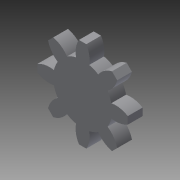
# Autodesk Inventor part: Planet
Saved by Autodesk Inventor 2013 (Build 170138000, 138)
## iProperties
Created: 2014-02-12
Part Number: Planet
Material: Generic
Document SubType Name: Modeling
Designer: robotics
Density: 1 g/cm^3
Author: robotics
Autodesk Inventor part; units mm, degrees
ref_plane "YZ Plane" through (0, 0, 0) normal (1, 0, 0) x (0, 1, 0)
ref_plane "XZ Plane" through (0, 0, 0) normal (0, 1, 0) x (-1, 0, 0)
ref_plane "XY Plane" through (0, 0, 0) normal (0, 0, 1) x (1, 0, 0)
sketch "Sketch2" plane through (0, 0, 0) normal (0, 0, 1) x (1, 0, 0)
  line L0 (0, 0) -> (0, 8.357) construction
  line L1 (0, 0) -> (2.8603, 0) construction
  arc A0 (-0.3969, 4.8591) -> (-0.71, 3.0831) centre (1.785, 3.5588) ccw
  arc A1 (0.71, 3.0831) -> (0.3969, 4.8591) centre (-1.785, 3.5588) ccw
  line L2 (0.3969, 4.8591) -> (-0.3969, 4.8591)
  line L3 (-0.71, 3.0831) -> (0.71, 3.0831) construction
  arc A2 (0.71, 3.0831) -> (0.3969, 4.8591) centre (-1.785, 3.5588) ccw
  line L4 (0.3969, 4.8591) -> (-0.3969, 4.8591)
  arc A3 (-0.3969, 4.8591) -> (-0.71, 3.0831) centre (1.785, 3.5588) ccw
  line L5 (0.3969, 4.8591) -> (0.71, 3.0831) construction
  arc A4 (-1.678, 2.6822) -> (-3.1553, 3.7166) centre (-3.7786, 1.2542) ccw
  line L6 (-3.1553, 3.7166) -> (-3.7166, 3.1553)
  arc A5 (-3.7166, 3.1553) -> (-2.6822, 1.678) centre (-1.2542, 3.7786) ccw
  arc A6 (-3.0831, 0.71) -> (-4.8591, 0.3969) centre (-3.5588, -1.785) ccw
  line L7 (-4.8591, 0.3969) -> (-4.8591, -0.3969)
  arc A7 (-4.8591, -0.3969) -> (-3.0831, -0.71) centre (-3.5588, 1.785) ccw
  arc A8 (-2.6822, -1.678) -> (-3.7166, -3.1553) centre (-1.2542, -3.7786) ccw
  line L8 (-3.7166, -3.1553) -> (-3.1553, -3.7166)
  arc A9 (-3.1553, -3.7166) -> (-1.678, -2.6822) centre (-3.7786, -1.2542) ccw
  arc A10 (-0.71, -3.0831) -> (-0.3969, -4.8591) centre (1.785, -3.5588) ccw
  line L9 (-0.3969, -4.8591) -> (0.3969, -4.8591)
  arc A11 (0.3969, -4.8591) -> (0.71, -3.0831) centre (-1.785, -3.5588) ccw
  arc A12 (1.678, -2.6822) -> (3.1553, -3.7166) centre (3.7786, -1.2542) ccw
  line L10 (3.1553, -3.7166) -> (3.7166, -3.1553)
  arc A13 (3.7166, -3.1553) -> (2.6822, -1.678) centre (1.2542, -3.7786) ccw
  arc A14 (3.0831, -0.71) -> (4.8591, -0.3969) centre (3.5588, 1.785) ccw
  line L11 (4.8591, -0.3969) -> (4.8591, 0.3969)
  arc A15 (4.8591, 0.3969) -> (3.0831, 0.71) centre (3.5588, -1.785) ccw
  arc A16 (2.6822, 1.678) -> (3.7166, 3.1553) centre (1.2542, 3.7786) ccw
  line L12 (3.7166, 3.1553) -> (3.1553, 3.7166)
  arc A17 (3.1553, 3.7166) -> (1.678, 2.6822) centre (3.7786, 1.2542) ccw
  line L13 (-1.678, 2.6822) -> (-0.71, 3.0831) construction
  arc A18 (-0.71, 3.0831) -> (-1.678, 2.6822) centre (0, 0) ccw
  arc A19 (1.678, 2.6822) -> (0.71, 3.0831) centre (0, 0) ccw
  arc A20 (3.0831, 0.71) -> (2.6822, 1.678) centre (0, 0) ccw
  arc A21 (2.6822, -1.678) -> (3.0831, -0.71) centre (0, 0) ccw
  arc A22 (0.71, -3.0831) -> (1.678, -2.6822) centre (0, 0) ccw
  arc A23 (-1.678, -2.6822) -> (-0.71, -3.0831) centre (0, 0) ccw
  arc A24 (-2.6822, 1.678) -> (-3.0831, 0.71) centre (0, 0) ccw
  arc A25 (-3.0831, -0.71) -> (-2.6822, -1.678) centre (0, 0) ccw
  point P0 (0, 4.8591)
  point P1 (-3.4359, 3.4359)
  point P2 (-4.8591, 0)
  point P3 (-3.4359, -3.4359)
  point P4 (0, -4.8591)
  point P5 (3.4359, -3.4359)
  point P6 (4.8591, 0)
  point P7 (3.4359, 3.4359)
  dimension "d11" = 0.7937
  dimension "d13" = 2.54
  dimension "d14" = 80
  dimension "d15" = 1.8034
  dimension "d18" = 360
  dimension "d20" = 1.0477
  constraints: 52 point on circle, 28 end point, 26 centre point, 2 concentric, 1 coincident, 1 collinear, 1 horizontal, 1 horizontal alignment, 1 midpoint, 1 parallel, 1 perpendicular, 1 vertical, 1 vertical alignment, 81 other
  measures "d11" distance of L2.start L2.end
  measures "d13" radius of A1
  measures "d14" angle of L1 L5
  measures "d15" distance of L2.start L3.end
  measures "d20" distance of L3.start L13.start
extrude "Extrusion2" add sketch "Sketch2" along normal blind 1.5875
body "Solid2"
